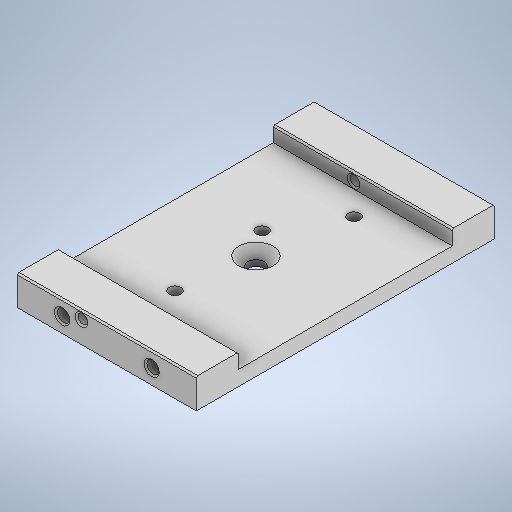
# Autodesk Inventor part: TS_V1_Fallmagazin_Wandung_int
Saved by Autodesk Inventor 2025.2 (Build 292293000, 293)
## iProperties
Created: 2025-06-10
Part Number: TS_V1_Fallmagazin_Wandung_int
Material: Generisch
Document SubType Name: Modeling
Designer: tino
Density: 1 g/cm^3
Appearance: Vorgabe
Author: tino
Autodesk Inventor part; units mm, degrees
ref_plane "YZ Plane" through (0, 0, 0) normal (1, 0, 0) x (0, 1, 0)
ref_plane "XZ Plane" through (0, 0, 0) normal (0, 1, 0) x (-1, 0, 0)
ref_plane "XY Plane" through (0, 0, 0) normal (0, 0, 1) x (1, 0, 0)
sketch "Skizze1" plane through (0, 0, 0) normal (0, 0, 1) x (1, 0, 0)
  arc A0 (-7.910725, 24.207043) -> (-7.910891, 20.407043) centre (-6.063513, 22.306962) ccw
  line L0 (-7.910725, 24.207043) -> (-4.216135, 24.206882)
  arc A1 (-4.216301, 20.406882) -> (-4.216135, 24.206882) centre (-6.063513, 22.306962) ccw
  line L1 (-4.216301, 20.406882) -> (-7.910891, 20.407043)
  spline S0 degree 3 poles (4.168227, 35.189684) (1.190462, 36.459804) (-2.249662, 35.164227) (-6.254955, 34.158153) (-11.73606, 32.147863) (-17.267484, 27.437) (-17.397864, 22.280527) (-19.179409, 11.837341) (-24.204265, -4.219772) (-21.912215, -21.361857) (-15.72629, -32.136108) (-8.960071, -34.873142) (-7.734356, -35.206805) knots 0 0 0 0 0.05534958 0.07652777 0.21178189 0.29554676 0.38296386 0.43292215 0.75488434 0.81234043 0.96723776 1 1 1 1
  spline S1 degree 3 poles (-7.734356, -35.206805) (-2.439109, -36.648242) (4.93418, -35.14496) (14.388893, -31.364077) (20.220621, -28.276552) (23.084745, -23.179223) (23.280953, -18.995872) (17.306215, -16.499664) (13.73981, -19.293705) (6.907357, -22.933236) (-1.198572, -27.162074) (-10.305482, -22.9326) (-14.035245, -10.40017) (-9.459871, -0.926027) (-6.833349, 0.315314) (-5.918232, 2.05884) (-5.936684, 4.17913) (-8.288714, 5.230646) (-8.364147, 10.437319) (-1.010592, 14.125066) (4.082108, 20.05073) (3.063503, 26.302613) (2.949283, 28.613576) (3.78883, 29.833993) (5.577793, 31.092404) (6.613193, 32.774527) (5.245759, 34.708646) (4.265654, 35.148112) (4.168227, 35.189684) knots 0 0 0 0 0.1415298 0.17035016 0.24598676 0.2589199 0.29022703 0.32626485 0.37223258 0.38897966 0.48209608 0.50825566 0.62441589 0.64741797 0.71527435 0.72606992 0.74689162 0.80172241 0.81188461 0.84851364 0.9163561 0.94337427 0.94821885 0.96295932 0.96650966 0.98187972 0.99818797 1 1 1 1
  line L2 (-4.216301, 20.406882) -> (-7.910891, 20.407043)
  arc A2 (-4.216301, 20.406882) -> (-4.216135, 24.206882) centre (-6.063513, 22.306962) ccw
  line L3 (-7.910725, 24.207043) -> (-4.216135, 24.206882)
  arc A3 (-7.910725, 24.207043) -> (-7.910891, 20.407043) centre (-6.063513, 22.306962) ccw
  line L4 (-22.994876, 35.829551) -> (22.994876, 35.829551) construction
  line L5 (22.994876, 35.829551) -> (22.994876, -35.829551) construction
  line L6 (22.994876, -35.829551) -> (-22.994876, -35.829551) construction
  line L7 (-22.994876, -35.829551) -> (-22.994876, 35.829551) construction
  line L8 (-22.994876, 35.829551) -> (22.994876, -35.829551) construction
  line L9 (-22.994876, -35.829551) -> (22.994876, 35.829551) construction
  circle A4 centre (3.874552, -36.279551) radius 1.25 construction
  line L10 (1.214575, -35.829551) -> (11.587679, -35.829551) construction
  line L11 (3.874552, -36.279551) -> (3.874552, -35.029551) construction
  circle A5 centre (4.795469, 36.279551) radius 1.25 construction
  line L12 (4.795469, 36.279551) -> (4.795469, 35.029551) construction
  line L13 (3.124047, 35.829551) -> (12.547009, 35.829551) construction
  point P0 (0, 0)
  point P1 (0, 0)
  point P2 (0, 0)
  dimension "d88" = 2.5
  dimension "d91" = 2.5
  dimension "d89" = 0.8
  dimension "d92" = 0.8
  constraints: 28 end point, 8 point on circle, 4 centre point, 4 perpendicular, 3 vertical, 2 collinear, 2 horizontal, 2 midpoint, 2 vertical alignment, 1 coincident, 8 other
sketch "Skizze9" plane through (0, 0, 0) normal (0, 0, 1) x (1, 0, 0)
  line L0 (-30, 46) -> (30, 46)
  line L1 (30, 46) -> (30, -46)
  line L2 (30, -46) -> (-30, -46)
  line L3 (-30, 46) -> (30, -46) construction
  line L4 (30, 46) -> (-30, -46) construction
  spline S0 degree 3 poles (4.168227, 35.189684) (1.190462, 36.459804) (-2.249662, 35.164227) (-6.254955, 34.158153) (-11.73606, 32.147863) (-17.267484, 27.437) (-17.397864, 22.280527) (-19.179409, 11.837341) (-24.204265, -4.219772) (-21.912215, -21.361857) (-15.72629, -32.136108) (-8.960071, -34.873142) (-7.734356, -35.206805) knots 0 0 0 0 0.05534958 0.07652777 0.21178189 0.29554676 0.38296386 0.43292215 0.75488434 0.81234043 0.96723776 1 1 1 1
  spline S1 degree 3 poles (-7.734356, -35.206805) (-2.439109, -36.648242) (4.93418, -35.14496) (14.388893, -31.364077) (20.220621, -28.276552) (23.084745, -23.179223) (23.280953, -18.995872) (17.306215, -16.499664) (13.73981, -19.293705) (6.907357, -22.933236) (-1.198572, -27.162074) (-10.305482, -22.9326) (-14.035245, -10.40017) (-9.459871, -0.926027) (-6.833349, 0.315314) (-5.918232, 2.05884) (-5.936684, 4.17913) (-8.288714, 5.230646) (-8.364147, 10.437319) (-1.010592, 14.125066) (4.082108, 20.05073) (3.063503, 26.302613) (2.949283, 28.613576) (3.78883, 29.833993) (5.577793, 31.092404) (6.613193, 32.774527) (5.245759, 34.708646) (4.265654, 35.148112) (4.168227, 35.189684) knots 0 0 0 0 0.1415298 0.17035016 0.24598676 0.2589199 0.29022703 0.32626485 0.37223258 0.38897966 0.48209608 0.50825566 0.62441589 0.64741797 0.71527435 0.72606992 0.74689162 0.80172241 0.81188461 0.84851364 0.9163561 0.94337427 0.94821885 0.96295932 0.96650966 0.98187972 0.99818797 1 1 1 1
  circle A0 centre (-3.5, -23.6754) radius 2
  circle A1 centre (5.000912, 27.85018) radius 2
  circle A2 centre (-6.3, 8.375362) radius 2
  line L5 (-30, -35.829553) -> (30, -35.829553)
  line L6 (-30, -46) -> (-30, 46)
  line L7 (-30, 35.829552) -> (30, 35.829552)
  point P0 (0, 0)
  point P1 (-2.781906, -35.829553)
  point P2 (1.073951, 35.829552)
  dimension "Laenge_aussen" = 105
  dimension "d68" = 60
  dimension "d69" = 92
  dimension "d180" = 4
  dimension "d182" = 4
  dimension "d183" = 4
  dimension "d184" = 33.5
  dimension "d186" = 24.99909
  dimension "d221" = 36.3
  constraints: 16 end point, 4 point on line, 3 centre point, 3 horizontal, 3 perpendicular, 2 midpoint, 1 parallel, 1 vertical, 4 other
  measures "d68" distance of L0.start L0.end
  measures "d69" distance of L0.end L1.end
  measures "d180" diameter of A0
  measures "d182" diameter of A2
  measures "d183" diameter of A1
  measures "d184" distance from line of L1 A0.centre
  measures "d186" distance from line of L1 A1.centre
  measures "d221" distance from line of L1 A2.centre
extrude "Extrusion3" add sketch "Skizze9" along normal blind 5 contours L0 L1 L7 L6 | L5 L1 L2 L6
sketch "Skizze11" plane through (0, 0, 0) normal (0, 0, -1) x (-1, 0, 0)
  line L0 (30, -46) -> (-30, -46) projected
  line L1 (30, 46) -> (30, -46) projected
  line L2 (-30, -46) -> (30, -46)
  line L3 (30, -46) -> (30, 46)
  line L4 (30, 46) -> (-30, 46)
  line L5 (-30, 46) -> (-30, -46)
  point P0 (0, 0)
  constraints: 8 end point, 2 parallel, 1 horizontal, 1 perpendicular
extrude "Extrusion4" add sketch "Skizze11" along normal blind 1.5
chamfer "Fasen2" distance 0.5 angle 45 2 edges at (0, -35.8296, 5) (0, 35.8296, 5)
sketch "Skizze15" plane through (-30, 46, 5) normal (0, 1, 0) x (1, 0, 0)
  line L0 (60, 0) -> (0, 0) projected
  line L1 (0, 6.5) -> (60, 6.5) projected
  line L2 (60, 0) -> (0, 0)
  line L3 (0, 0) -> (0, 6.5)
  line L4 (0, 6.5) -> (60, 6.5)
  line L5 (60, 6.5) -> (60, 0)
  point P0 (30, 5)
  constraints: 8 end point, 2 parallel, 1 horizontal, 1 perpendicular
extrude "Extrusion6" add sketch "Skizze15" along normal blind 4
sketch "Skizze16" plane through (-30, -46, 5) normal (0, -1, 0) x (1, 0, 0)
  line L0 (0, -6.5) -> (0, 0) projected
  line L1 (60, -6.5) -> (0, -6.5) projected
  line L2 (0, 0) -> (60, 0)
  line L3 (60, 0) -> (60, -6.5)
  line L4 (60, -6.5) -> (0, -6.5)
  line L5 (0, -6.5) -> (0, 0)
  point P0 (30, -5)
  constraints: 8 end point, 2 parallel, 1 horizontal, 1 perpendicular
extrude "Extrusion7" add sketch "Skizze16" along normal blind 4
sketch "Skizze17" plane through (0, 0, -1.5) normal (0, 0, -1) x (-1, 0, 0)
  line L0 (30, 50) -> (30, -50) projected
  line L1 (-30, 50) -> (30, 50) projected
  line L2 (-30, -50) -> (-30, 50) projected
  line L3 (30, -50) -> (-30, -50) projected
  point P0 (0, 0)
extrude "Extrusion8" add sketch "Skizze17" along normal blind 3.5
chamfer "Fasen4" distance 0.5 angle 45 2 edges at (0, 50, 5) (0, -50, 5)
sketch "Skizze20" plane through (0, 0, 0) normal (0, 0, 1) x (1, 0, 0)
  line L0 (-30, -50) -> (30, -50)
  line L1 (30, 35.829552) -> (30, -35.829553)
  point P0 (0, 0)
  point P1 (-30, -46.5)
  point P2 (0, 0)
  constraints: 1 other
hole "Bohrung10" at (0, 0, 0) direction (0, 0, -1) diameter 5.5 end through all countersink diameter 11.5 countersink angle 90
sketch "Skizze21" plane through (-30, -50, 5) normal (0, -1, 0) x (1, 0, 0)
  line L0 (60, -10) -> (0, -10) projected
  line L1 (60, 0) -> (0, 0) projected
  line L2 (60, -0.5) -> (60, -10) projected
  line L3 (0, -0.5) -> (0, -10) projected
  point P0 (30, -5)
  point P1 (15, -5)
  point P2 (45, -5)
  point P3 (60, -5.25)
  dimension "d161" = 10
  dimension "d163" = 60
  dimension "d164" = 15
  dimension "d165" = 15
  dimension "d179" = 5
  constraints: 1 horizontal alignment, 1 midpoint
  measures "d161" distance between parallel lines of L0 L1
  measures "d163" distance between parallel lines of L2 L3
  measures "d164" distance from line of L3 point (15, -5)
  measures "d165" horizontal distance of point (60, -5.25) point (45, -5)
  measures "d179" distance from line of L0 point (15, -5)
hole "Bohrung11" at (15, -50, 0) at (-15, -50, 0) direction (0, 1, 0) diameter 4.134 depth 6 tip angle 118 thread size "M5x0.8" class "6H" standard "ISO Metric profile"
chamfer "Fasen5" distance 0.5 angle 45 2 edges at (-15, -50, 2.067) (15, -50, 2.067)
mirror "Spiegeln4" about plane through (0, 0, 0) normal (0, 1, 0) of "Bohrung11"
chamfer "Fasen6" distance 0.5 angle 45 2 edges at (15, 50, 2.067) (-15, 50, 2.067)
sketch "Skizze22" plane through (0, 0, 0) normal (0, 0, 1) x (1, 0, 0)
  circle A0 centre (-8.52675, -36.279553) radius 1.25 construction
  line L0 (30, -35.829553) -> (-30, -35.829553) construction
  line L1 (-19.029206, -35.029553) -> (-13.234121, -35.029553) construction
  spline S0 degree 3 poles (4.168227, 35.189684) (1.190462, 36.459804) (-2.249662, 35.164227) (-6.254955, 34.158153) (-11.73606, 32.147863) (-17.267484, 27.437) (-17.397864, 22.280527) (-19.179409, 11.837341) (-24.204265, -4.219772) (-21.912215, -21.361857) (-15.72629, -32.136108) (-8.960071, -34.873142) (-7.734356, -35.206805) knots 0 0 0 0 0.05534958 0.07652777 0.21178189 0.29554676 0.38296386 0.43292215 0.75488434 0.81234043 0.96723776 1 1 1 1 construction
  circle A1 centre (-3.073907, 36.279552) radius 1.25 construction
  line L2 (-18.70543, 35.029552) -> (-14.396256, 35.029552) construction
  line L3 (-30, 35.829552) -> (30, 35.829552) construction
  point P0 (0, 0)
  dimension "d188" = 2.5
  dimension "d189" = 0.8
  dimension "d190" = 2.5
  dimension "d191" = 0.8
  constraints: 4 end point, 2 centre point, 2 horizontal, 2 tangent, 2 other
  measures "d188" diameter of A0
  measures "d189" distance between parallel lines of L0 L1
  measures "d190" diameter of A1
  measures "d191" distance between parallel lines of L3 L2
sketch "Skizze23" plane through (-30, -35.829553, 0) normal (0, 1, 0) x (1, 0, 0)
  line L0 (20.22325, 0) -> (22.72325, 0) construction
  line L1 (0, -5) -> (60, -5)
  line L2 (60, -4.5) -> (0, -4.5)
  line L3 (60, 0) -> (0, 0)
  point P0 (30, 0)
  point P1 (21.47325, -2.25)
  point P2 (21.47325, 0)
  dimension "d218" = 4.5
  dimension "d219" = 2.25
  constraints: 1 midpoint, 1 vertical alignment
  measures "d218" distance between parallel lines of L2 L3
  measures "d219" distance from line of L3 point (21.473, -2.25)
hole "Bohrung12" at (-8.52675, -35.829553, 2.25) direction (0, -1, 0) diameter 3.242 end through all thread size "M4x0.7" class "6H" standard "ISO Metric profile"
chamfer "Fasen7" distance 0.5 angle 45 2 edges at (-8.5267, -35.8296, 0.629) (-8.5267, -50, 0.629)
sketch "Skizze24" plane through (-30, 35.829552, 0) normal (0, -1, 0) x (1, 0, 0)
  line L0 (28.176093, 0) -> (25.676093, 0) construction
  line L1 (60, 5) -> (0, 5)
  line L2 (0, 0) -> (60, 0)
  line L3 (0, 4.5) -> (60, 4.5)
  point P0 (30, 0)
  point P1 (26.926093, 2.25)
  point P2 (26.926093, 0)
  dimension "d205" = 2.25
  dimension "d220" = 4.5
  constraints: 1 midpoint, 1 vertical alignment
  measures "d205" distance from line of point (26.926, 2.25) L2
  measures "d220" distance between parallel lines of L3 L2
hole "Bohrung13" at (-3.073907, 35.829552, 2.25) direction (0, 1, 0) diameter 3.242 end through all thread size "M4x0.7" class "6H" standard "ISO Metric profile"
chamfer "Fasen8" distance 0.5 angle 45 2 edges at (-3.0739, 35.8296, 3.871) (-3.0739, 50, 3.871)
extrude "Extrusion10" cut sketch "Skizze9" against normal blind 3 contours A0 | A2 | A1
equation "\"d91\" = Kugeldurchmesser"
equation "\"d89\" = Kugelhoehe"
equation "\"d92\" = Kugelhoehe"
equation "\"Laenge_aussen\" = Laenge_innen + 2 * Wanddicke"
equation "\"d68\" = Breite_innen"
equation "\"d191\" = d189"
equation "\"Breite_innen\" = 60"
equation "\"Laenge_innen\" = 85"
equation "\"Absatz\" = 2"
equation "\"Kugeldurchmesser\" = 2.5"
equation "\"Kugelhoehe\" = 0.8"
equation "\"Anbindung_Kolben\" = 15"
equation "\"Wanddicke\" = 10"
